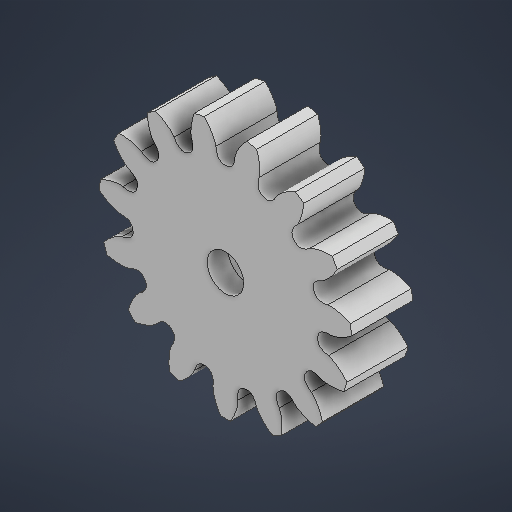
# Autodesk Inventor part: sg90 claw v2 gear m1
Saved by Autodesk Inventor 2026.1 (Build 301233020, 233B)
## iProperties
Created: 2025-05-11
Part Number: sg90 claw v2 gear m1
Material: Generic
Document SubType Name: Modeling
Designer: gavin
Density: 1 g/cm^3
Appearance: Default
Author: gavin
## iProperties of the stored document sg90 claw v2 gear m1_3D 列印.ipt
Created: 2025-05-11
Part Number: sg90 claw v2 gear m1_3D 列印
Material: 一般
Document SubType Name: Modeling
Designer: gavin
Density: 1 g/cm^3
Appearance: 預設
Author: gavin
Autodesk Inventor part; units mm, degrees
(part 1 of 2)
ref_plane "YZ Plane" through (0, 0, 0) normal (1, 0, 0) x (0, 1, 0)
ref_plane "XZ Plane" through (0, 0, 0) normal (0, 1, 0) x (-1, 0, 0)
ref_plane "XY Plane" through (0, 0, 0) normal (0, 0, 1) x (1, 0, 0)
sketch "Sketch1" plane through (0, 0, 0) normal (0, 0, 1) x (1, 0, 0)
  spline S0 degree 3 poles (-1.4265, 8.3497) (-1.3822, 8.3018) (-1.2937, 8.2061) (-1.1693, 8.0552) (-1.0517, 7.8988) (-0.9427, 7.7364) (-0.8433, 7.568) (-0.7701, 7.4222) (-0.7188, 7.3023) (-0.6849, 7.2106) (-0.6553, 7.1173) (-0.6433, 7.0532) (-0.6374, 7.0212) knots 0 0 0 0 0.125009 0.250019 0.375027 0.500033 0.625034 0.750026 0.812532 0.875035 0.937534 1 1 1 1
  spline S1 degree 3 poles (-0.6374, 7.0212) (-0.6343, 6.9735) (-0.6298, 6.9019) (-0.6162, 6.8071) (-0.6007, 6.7371) (-0.5816, 6.6679) (-0.5564, 6.6007) (-0.527, 6.5352) (-0.4905, 6.4733) (-0.4477, 6.4156) (-0.3983, 6.3633) (-0.3422, 6.3182) (-0.2804, 6.2814) (-0.2136, 6.2546) (-0.1435, 6.2382) (-0.0717, 6.2343) (0, 6.2359) (0.0717, 6.2343) (0.1435, 6.2382) (0.2136, 6.2546) (0.2804, 6.2814) (0.3422, 6.3182) (0.3983, 6.3633) (0.4477, 6.4156) (0.4905, 6.4733) (0.527, 6.5352) (0.5564, 6.6007) (0.5816, 6.6679) (0.6007, 6.7371) (0.6162, 6.8071) (0.6298, 6.9019) (0.6343, 6.9735) (0.6374, 7.0212) knots 0 0 0 0 0.062496 0.093751 0.125009 0.156269 0.187518 0.218773 0.250034 0.281288 0.312536 0.343783 0.375036 0.406281 0.437514 0.468742 0.5 0.531258 0.562486 0.593719 0.624964 0.656217 0.687464 0.718712 0.749966 0.781227 0.812482 0.843731 0.874991 0.906249 0.937504 1 1 1 1
  spline S2 degree 3 poles (0.6374, 7.0212) (0.6433, 7.0532) (0.6553, 7.1173) (0.6849, 7.2106) (0.7188, 7.3023) (0.7701, 7.4222) (0.8433, 7.568) (0.9427, 7.7364) (1.0517, 7.8988) (1.1693, 8.0552) (1.2937, 8.2061) (1.3822, 8.3018) (1.4265, 8.3497) knots 0 0 0 0 0.062466 0.124965 0.187468 0.249974 0.374966 0.499967 0.624973 0.749981 0.874991 1 1 1 1
  circle A0 centre (0, 0) radius 6.2354 construction
  circle A1 centre (0, 0) radius 7.0477 construction
  circle A2 centre (0, 0) radius 7.5 construction
  circle A3 centre (0, 0) radius 8.4706
  point P0 (-1.2951, 8.2049)
  point P1 (-1.1704, 8.0543)
  point P2 (-1.0532, 7.8978)
  point P3 (-0.9443, 7.7354)
  point P4 (-0.8452, 7.5669)
  point P5 (-0.7579, 7.392)
  point P6 (-0.7196, 7.302)
  point P7 (-0.6856, 7.2104)
  point P8 (-0.6572, 7.1168)
  point P9 (-0.6258, 6.8783)
  point P10 (-0.6153, 6.8073)
  point P11 (-0.6001, 6.7372)
  point P12 (-0.5806, 6.6682)
  point P13 (-0.5557, 6.6009)
  point P14 (-0.5258, 6.5358)
  point P15 (-0.4894, 6.4739)
  point P16 (-0.4466, 6.4165)
  point P17 (-0.3972, 6.3645)
  point P18 (-0.3413, 6.3196)
  point P19 (-0.2795, 6.2831)
  point P20 (-0.213, 6.2563)
  point P21 (-0.1432, 6.2403)
  point P22 (-0.0717, 6.2352)
  point P23 (0, 6.2354)
  point P24 (0.0717, 6.2352)
  point P25 (0.1432, 6.2403)
  point P26 (0.213, 6.2563)
  point P27 (0.2795, 6.2831)
  point P28 (0.3413, 6.3196)
  point P29 (0.3972, 6.3645)
  point P30 (0.4466, 6.4165)
  point P31 (0.4894, 6.4739)
  point P32 (0.5258, 6.5358)
  point P33 (0.5557, 6.6009)
  point P34 (0.5806, 6.6682)
  point P35 (0.6001, 6.7372)
  point P36 (0.6153, 6.8073)
  point P37 (0.6258, 6.8783)
  point P38 (0.6572, 7.1168)
  point P39 (0.6856, 7.2104)
  point P40 (0.7196, 7.302)
  point P41 (0.7579, 7.392)
  point P42 (0.8452, 7.5669)
  point P43 (0.9443, 7.7354)
  point P44 (1.0532, 7.8978)
  point P45 (1.1704, 8.0543)
  point P46 (1.2951, 8.2049)
  constraints: 4 centre point, 2 point on circle, 109 other
extrude "擠出1" add sketch "Sketch1" against normal blind 2.7
extrude "擠出2" cut sketch "Sketch1" against normal through all contours A3 S2 S1 S0 picked at (0.1465, 7.7452)
pattern_circular "環形陣列1" count 15 over 360 about axis through (0, 0, -10) along (0, 0, 1) of "擠出2"
sketch "草圖2" plane through (0, 0, 0) normal (0, 0, 1) x (1, 0, 0)
  circle A0 centre (0, 0) radius 2.2975
  dimension "d7" = 4.595
  constraints: 1 centre point, 1 coincident
  measures "d7" diameter of A0
extrude "擠出3" cut sketch "草圖2" against normal through all
sketch "草圖3" plane through (0, 0, 0) normal (0, 0, 1) x (1, 0, 0)
  circle A0 centre (0, 0) radius 2.2975 projected
  spline S0 degree 3 poles (4.6993, 7.0476) (4.6394, 7.0219) (4.5196, 6.9704) (4.3445, 6.8832) (4.1736, 6.7882) (4.0079, 6.6842) (3.8485, 6.5707) (3.7224, 6.4673) (3.6268, 6.3787) (3.5586, 6.3087) (3.4935, 6.2355) (3.4565, 6.1818) (3.438, 6.1549) knots 0 0 0 0 0.125009 0.250019 0.375027 0.500033 0.625034 0.750026 0.812532 0.875035 0.937534 1 1 1 1 projected
  spline S1 degree 3 poles (3.438, 6.1549) (3.4159, 6.1126) (3.3826, 6.049) (3.3316, 5.968) (3.289, 5.9103) (3.2434, 5.8548) (3.193, 5.8037) (3.1395, 5.7558) (3.081, 5.7141) (3.0184, 5.6788) (2.952, 5.6512) (2.8825, 5.6328) (2.811, 5.6244) (2.7391, 5.627) (2.6684, 5.6405) (2.6012, 5.6662) (2.5364, 5.6968) (2.4702, 5.7245) (2.4062, 5.7572) (2.3488, 5.8007) (2.2988, 5.8524) (2.2572, 5.9112) (2.2244, 5.9752) (2.2005, 6.043) (2.1848, 6.1131) (2.1766, 6.1845) (2.1764, 6.2563) (2.1807, 6.328) (2.1915, 6.3989) (2.2058, 6.4693) (2.2319, 6.5613) (2.2569, 6.6286) (2.2735, 6.6734) knots 0 0 0 0 0.062496 0.093751 0.125009 0.156269 0.187518 0.218773 0.250034 0.281288 0.312536 0.343783 0.375036 0.406281 0.437514 0.468742 0.5 0.531258 0.562486 0.593719 0.624964 0.656217 0.687464 0.718712 0.749966 0.781227 0.812482 0.843731 0.874991 0.906249 0.937504 1 1 1 1 projected
  spline S2 degree 3 poles (2.2735, 6.6734) (2.2811, 6.7051) (2.2963, 6.7685) (2.3071, 6.8658) (2.3135, 6.9634) (2.3154, 7.0938) (2.3078, 7.2567) (2.2855, 7.451) (2.2519, 7.6437) (2.2081, 7.8343) (2.1559, 8.0228) (2.1139, 8.1463) (2.093, 8.208) knots 0 0 0 0 0.062466 0.124965 0.187468 0.249974 0.374966 0.499967 0.624973 0.749981 0.874991 1 1 1 1 projected
  arc A1 (2.093, 8.208) -> (1.4265, 8.3497) centre (0, 0) ccw projected
  spline S3 degree 3 poles (1.4265, 8.3497) (1.3822, 8.3018) (1.2937, 8.2061) (1.1693, 8.0552) (1.0517, 7.8988) (0.9427, 7.7364) (0.8433, 7.568) (0.7701, 7.4222) (0.7188, 7.3023) (0.6849, 7.2106) (0.6553, 7.1173) (0.6433, 7.0532) (0.6374, 7.0212) knots 0 0 0 0 0.125009 0.250019 0.375027 0.500033 0.625034 0.750026 0.812532 0.875035 0.937534 1 1 1 1 projected
  spline S4 degree 3 poles (0.6374, 7.0212) (0.6343, 6.9735) (0.6298, 6.9019) (0.6162, 6.8071) (0.6007, 6.7371) (0.5816, 6.6679) (0.5564, 6.6007) (0.527, 6.5352) (0.4905, 6.4733) (0.4477, 6.4156) (0.3983, 6.3633) (0.3422, 6.3182) (0.2804, 6.2814) (0.2136, 6.2546) (0.1435, 6.2382) (0.0717, 6.2343) (0, 6.2359) (-0.0717, 6.2343) (-0.1435, 6.2382) (-0.2136, 6.2546) (-0.2804, 6.2814) (-0.3422, 6.3182) (-0.3983, 6.3633) (-0.4477, 6.4156) (-0.4905, 6.4733) (-0.527, 6.5352) (-0.5564, 6.6007) (-0.5816, 6.6679) (-0.6007, 6.7371) (-0.6162, 6.8071) (-0.6298, 6.9019) (-0.6343, 6.9735) (-0.6374, 7.0212) knots 0 0 0 0 0.062496 0.093751 0.125009 0.156269 0.187518 0.218773 0.250034 0.281288 0.312536 0.343783 0.375036 0.406281 0.437514 0.468742 0.5 0.531258 0.562486 0.593719 0.624964 0.656217 0.687464 0.718712 0.749966 0.781227 0.812482 0.843731 0.874991 0.906249 0.937504 1 1 1 1 projected
  spline S5 degree 3 poles (-0.6374, 7.0212) (-0.6433, 7.0532) (-0.6553, 7.1173) (-0.6849, 7.2106) (-0.7188, 7.3023) (-0.7701, 7.4222) (-0.8433, 7.568) (-0.9427, 7.7364) (-1.0517, 7.8988) (-1.1693, 8.0552) (-1.2937, 8.2061) (-1.3822, 8.3018) (-1.4265, 8.3497) knots 0 0 0 0 0.062466 0.124965 0.187468 0.249974 0.374966 0.499967 0.624973 0.749981 0.874991 1 1 1 1 projected
  arc A2 (-1.4265, 8.3497) -> (-2.093, 8.208) centre (0, 0) ccw projected
  spline S6 degree 3 poles (-2.093, 8.208) (-2.1139, 8.1463) (-2.1559, 8.0228) (-2.2081, 7.8343) (-2.2519, 7.6437) (-2.2855, 7.451) (-2.3078, 7.2567) (-2.3154, 7.0938) (-2.3135, 6.9634) (-2.3071, 6.8658) (-2.2963, 6.7685) (-2.2811, 6.7051) (-2.2735, 6.6734) knots 0 0 0 0 0.125009 0.250019 0.375027 0.500033 0.625034 0.750026 0.812532 0.875035 0.937534 1 1 1 1 projected
  spline S7 degree 3 poles (-2.2735, 6.6734) (-2.2569, 6.6286) (-2.2319, 6.5613) (-2.2058, 6.4693) (-2.1915, 6.3989) (-2.1807, 6.328) (-2.1764, 6.2563) (-2.1766, 6.1845) (-2.1848, 6.1131) (-2.2005, 6.043) (-2.2244, 5.9752) (-2.2572, 5.9112) (-2.2988, 5.8524) (-2.3488, 5.8007) (-2.4062, 5.7572) (-2.4702, 5.7245) (-2.5364, 5.6968) (-2.6012, 5.6662) (-2.6684, 5.6405) (-2.7391, 5.627) (-2.811, 5.6244) (-2.8825, 5.6328) (-2.952, 5.6512) (-3.0184, 5.6788) (-3.081, 5.7141) (-3.1395, 5.7558) (-3.193, 5.8037) (-3.2434, 5.8548) (-3.289, 5.9103) (-3.3316, 5.968) (-3.3826, 6.049) (-3.4159, 6.1126) (-3.438, 6.1549) knots 0 0 0 0 0.062496 0.093751 0.125009 0.156269 0.187518 0.218773 0.250034 0.281288 0.312536 0.343783 0.375036 0.406281 0.437514 0.468742 0.5 0.531258 0.562486 0.593719 0.624964 0.656217 0.687464 0.718712 0.749966 0.781227 0.812482 0.843731 0.874991 0.906249 0.937504 1 1 1 1 projected
  spline S8 degree 3 poles (-3.438, 6.1549) (-3.4565, 6.1818) (-3.4935, 6.2355) (-3.5586, 6.3087) (-3.6268, 6.3787) (-3.7224, 6.4673) (-3.8485, 6.5707) (-4.0079, 6.6842) (-4.1736, 6.7882) (-4.3445, 6.8832) (-4.5196, 6.9704) (-4.6394, 7.0219) (-4.6993, 7.0476) knots 0 0 0 0 0.062466 0.124965 0.187468 0.249974 0.374966 0.499967 0.624973 0.749981 0.874991 1 1 1 1 projected
  arc A3 (-4.6993, 7.0476) -> (-5.2505, 6.6471) centre (0, 0) ccw projected
  spline S9 degree 3 poles (-5.2505, 6.6471) (-5.2446, 6.5822) (-5.2327, 6.4524) (-5.2037, 6.2589) (-5.1662, 6.0669) (-5.1185, 5.8772) (-5.0598, 5.6906) (-5.0005, 5.5387) (-4.9457, 5.4204) (-4.9002, 5.3339) (-4.8508, 5.2494) (-4.8111, 5.1976) (-4.7913, 5.1717) knots 0 0 0 0 0.125009 0.250019 0.375027 0.500033 0.625034 0.750026 0.812532 0.875035 0.937534 1 1 1 1 projected
  spline S10 degree 3 poles (-4.7913, 5.1717) (-4.7578, 5.1376) (-4.7077, 5.0863) (-4.6464, 5.0128) (-4.6047, 4.9544) (-4.566, 4.8939) (-4.5329, 4.8302) (-4.5039, 4.7645) (-4.4824, 4.696) (-4.4681, 4.6255) (-4.4624, 4.5539) (-4.4663, 4.482) (-4.4804, 4.4115) (-4.5051, 4.3439) (-4.5399, 4.2808) (-4.585, 4.2248) (-4.6342, 4.1726) (-4.6809, 4.1183) (-4.7319, 4.0675) (-4.791, 4.0264) (-4.8556, 3.9948) (-4.9243, 3.9734) (-4.9954, 3.9619) (-5.0672, 3.9602) (-5.1388, 3.9669) (-5.2092, 3.9812) (-5.2776, 4.0032) (-5.3444, 4.0294) (-5.4086, 4.0616) (-5.471, 4.0969) (-5.5505, 4.1502) (-5.6067, 4.1947) (-5.6442, 4.2244) knots 0 0 0 0 0.062496 0.093751 0.125009 0.156269 0.187518 0.218773 0.250034 0.281288 0.312536 0.343783 0.375036 0.406281 0.437514 0.468742 0.5 0.531258 0.562486 0.593719 0.624964 0.656217 0.687464 0.718712 0.749966 0.781227 0.812482 0.843731 0.874991 0.906249 0.937504 1 1 1 1 projected
  spline S11 degree 3 poles (-5.6442, 4.2244) (-5.672, 4.2414) (-5.7277, 4.2755) (-5.8169, 4.3159) (-5.9077, 4.3521) (-6.0311, 4.3941) (-6.1884, 4.4373) (-6.3801, 4.4761) (-6.5737, 4.5038) (-6.7685, 4.521) (-6.964, 4.5295) (-7.0943, 4.5278) (-7.1595, 4.5269) knots 0 0 0 0 0.062466 0.124965 0.187468 0.249974 0.374966 0.499967 0.624973 0.749981 0.874991 1 1 1 1 projected
  arc A4 (-7.1595, 4.5269) -> (-7.5002, 3.9369) centre (0, 0) ccw projected
  spline S12 degree 3 poles (-7.5002, 3.9369) (-7.4684, 3.88) (-7.4047, 3.7662) (-7.2996, 3.6012) (-7.1872, 3.4411) (-7.0665, 3.2872) (-6.937, 3.1406) (-6.821, 3.026) (-6.7228, 2.9402) (-6.6461, 2.8796) (-6.5665, 2.8226) (-6.5092, 2.7914) (-6.4806, 2.7758) knots 0 0 0 0 0.125009 0.250019 0.375027 0.500033 0.625034 0.750026 0.812532 0.875035 0.937534 1 1 1 1 projected
  spline S13 degree 3 poles (-6.4806, 2.7758) (-6.4361, 2.7582) (-6.3694, 2.7318) (-6.2836, 2.6896) (-6.2217, 2.6532) (-6.1618, 2.6137) (-6.1057, 2.5689) (-6.0524, 2.5207) (-6.0049, 2.4668) (-5.9632, 2.4083) (-5.9288, 2.3451) (-5.9032, 2.2779) (-5.8874, 2.2077) (-5.8825, 2.1359) (-5.8885, 2.0642) (-5.907, 1.9947) (-5.9307, 1.927) (-5.9513, 1.8583) (-5.9772, 1.7912) (-6.0145, 1.7296) (-6.0606, 1.6744) (-6.1147, 1.6269) (-6.1749, 1.5876) (-6.2399, 1.5568) (-6.308, 1.5339) (-6.3782, 1.5182) (-6.4495, 1.5105) (-6.5213, 1.5073) (-6.593, 1.5106) (-6.6644, 1.5175) (-6.7587, 1.5338) (-6.8282, 1.5516) (-6.8745, 1.5635) knots 0 0 0 0 0.062496 0.093751 0.125009 0.156269 0.187518 0.218773 0.250034 0.281288 0.312536 0.343783 0.375036 0.406281 0.437514 0.468742 0.5 0.531258 0.562486 0.593719 0.624964 0.656217 0.687464 0.718712 0.749966 0.781227 0.812482 0.843731 0.874991 0.906249 0.937504 1 1 1 1 projected
  spline S14 degree 3 poles (-6.8745, 1.5635) (-6.9068, 1.5677) (-6.9715, 1.5762) (-7.0694, 1.5768) (-7.1671, 1.5729) (-7.2969, 1.5612) (-7.4581, 1.5366) (-7.6491, 1.4941) (-7.8372, 1.4406) (-8.0222, 1.3771) (-8.2042, 1.3054) (-8.3226, 1.2508) (-8.3818, 1.2235) knots 0 0 0 0 0.062466 0.124965 0.187468 0.249974 0.374966 0.499967 0.624973 0.749981 0.874991 1 1 1 1 projected
  arc A5 (-8.3818, 1.2235) -> (-8.453, 0.5459) centre (0, 0) ccw projected
  spline S15 degree 3 poles (-8.453, 0.5459) (-8.4008, 0.5069) (-8.2964, 0.4288) (-8.1333, 0.3209) (-7.9655, 0.2203) (-7.7926, 0.1289) (-7.6146, 0.0476) (-7.4621, -0.0099) (-7.3375, -0.0484) (-7.2427, -0.0725) (-7.1468, -0.0923) (-7.0818, -0.0975) (-7.0493, -0.1) knots 0 0 0 0 0.125009 0.250019 0.375027 0.500033 0.625034 0.750026 0.812532 0.875035 0.937534 1 1 1 1 projected
  spline S16 degree 3 poles (-7.0493, -0.1) (-7.0016, -0.0981) (-6.9299, -0.0951) (-6.8343, -0.0987) (-6.763, -0.1068) (-6.6921, -0.1185) (-6.6227, -0.1366) (-6.5544, -0.159) (-6.4891, -0.1888) (-6.4272, -0.2254) (-6.3701, -0.2691) (-6.3194, -0.3201) (-6.2763, -0.3778) (-6.2427, -0.4413) (-6.219, -0.5094) (-6.2076, -0.5804) (-6.2018, -0.6518) (-6.1927, -0.7229) (-6.189, -0.7948) (-6.198, -0.8662) (-6.2177, -0.9354) (-6.2478, -1.0008) (-6.2868, -1.0612) (-6.3336, -1.1158) (-6.3865, -1.1644) (-6.4443, -1.2072) (-6.5063, -1.2433) (-6.5705, -1.2754) (-6.6374, -1.3016) (-6.7054, -1.3244) (-6.7982, -1.3478) (-6.8689, -1.3598) (-6.9161, -1.3678) knots 0 0 0 0 0.062496 0.093751 0.125009 0.156269 0.187518 0.218773 0.250034 0.281288 0.312536 0.343783 0.375036 0.406281 0.437514 0.468742 0.5 0.531258 0.562486 0.593719 0.624964 0.656217 0.687464 0.718712 0.749966 0.781227 0.812482 0.843731 0.874991 0.906249 0.937504 1 1 1 1 projected
  spline S17 degree 3 poles (-6.9161, -1.3678) (-6.9473, -1.3771) (-7.0099, -1.3956) (-7.0995, -1.4349) (-7.1872, -1.4782) (-7.3011, -1.5417) (-7.4383, -1.6297) (-7.5955, -1.7462) (-7.7456, -1.8716) (-7.8888, -2.0049) (-8.0259, -2.1444) (-8.1118, -2.2424) (-8.1548, -2.2914) knots 0 0 0 0 0.062466 0.124965 0.187468 0.249974 0.374966 0.499967 0.624973 0.749981 0.874991 1 1 1 1 projected
  arc A6 (-8.1548, -2.2914) -> (-7.9443, -2.9395) centre (0, 0) ccw projected
  spline S18 degree 3 poles (-7.9443, -2.9395) (-7.8807, -2.9539) (-7.7535, -2.9827) (-7.5606, -3.015) (-7.3665, -3.0386) (-7.1713, -3.0518) (-6.9757, -3.0537) (-6.8129, -3.0442) (-6.6834, -3.0287) (-6.5871, -3.0121) (-6.4914, -2.9912) (-6.4299, -2.9695) (-6.3992, -2.9586) knots 0 0 0 0 0.125009 0.250019 0.375027 0.500033 0.625034 0.750026 0.812532 0.875035 0.937534 1 1 1 1 projected
  spline S19 degree 3 poles (-6.3992, -2.9586) (-6.3564, -2.9374) (-6.2921, -2.9055) (-6.2033, -2.8699) (-6.1348, -2.8483) (-6.0654, -2.8302) (-5.9945, -2.8185) (-5.9231, -2.8112) (-5.8512, -2.8119) (-5.7799, -2.8201) (-5.7099, -2.8368) (-5.6428, -2.8627) (-5.5801, -2.8979) (-5.5234, -2.9423) (-5.4742, -2.9948) (-5.4349, -3.0551) (-5.4005, -3.118) (-5.3632, -3.1792) (-5.3307, -3.2433) (-5.3098, -3.3123) (-5.2997, -3.3835) (-5.3006, -3.4555) (-5.3117, -3.5266) (-5.3322, -3.5955) (-5.3608, -3.6614) (-5.3961, -3.724) (-5.4381, -3.7822) (-5.4837, -3.8376) (-5.5341, -3.8887) (-5.5871, -3.9372) (-5.6623, -3.9964) (-5.722, -4.0361) (-5.7618, -4.0626) knots 0 0 0 0 0.062496 0.093751 0.125009 0.156269 0.187518 0.218773 0.250034 0.281288 0.312536 0.343783 0.375036 0.406281 0.437514 0.468742 0.5 0.531258 0.562486 0.593719 0.624964 0.656217 0.687464 0.718712 0.749966 0.781227 0.812482 0.843731 0.874991 0.906249 0.937504 1 1 1 1 projected
  spline S20 degree 3 poles (-5.7618, -4.0626) (-5.7866, -4.0838) (-5.8362, -4.1261) (-5.9021, -4.1985) (-5.9646, -4.2737) (-6.0428, -4.378) (-6.1324, -4.5143) (-6.2286, -4.6846) (-6.3147, -4.8603) (-6.3913, -5.0402) (-6.4598, -5.2234) (-6.4985, -5.3479) (-6.5178, -5.4102) knots 0 0 0 0 0.062466 0.124965 0.187468 0.249974 0.374966 0.499967 0.624973 0.749981 0.874991 1 1 1 1 projected
  arc A7 (-6.5178, -5.4102) -> (-6.0619, -5.9166) centre (0, 0) ccw projected
  spline S21 degree 3 poles (-6.0619, -5.9166) (-5.9979, -5.9039) (-5.8701, -5.8785) (-5.6807, -5.8295) (-5.4937, -5.7721) (-5.31, -5.7048) (-5.1306, -5.6269) (-4.9857, -5.552) (-4.8737, -5.4852) (-4.7924, -5.4309) (-4.7136, -5.3729) (-4.6662, -5.328) (-4.6426, -5.3056) knots 0 0 0 0 0.125009 0.250019 0.375027 0.500033 0.625034 0.750026 0.812532 0.875035 0.937534 1 1 1 1 projected
  spline S22 degree 3 poles (-4.6426, -5.3056) (-4.6121, -5.2688) (-4.5663, -5.2135) (-4.4997, -5.1449) (-4.4459, -5.0973) (-4.3898, -5.0525) (-4.3299, -5.013) (-4.2676, -4.9773) (-4.2017, -4.9487) (-4.1331, -4.9272) (-4.0625, -4.9139) (-3.9906, -4.9104) (-3.919, -4.917) (-3.8492, -4.9345) (-3.7828, -4.9625) (-3.7224, -5.0015) (-3.6654, -5.045) (-3.6064, -5.0858) (-3.5506, -5.1311) (-3.5035, -5.1856) (-3.4653, -5.2466) (-3.4369, -5.3127) (-3.4181, -5.3821) (-3.4088, -5.4534) (-3.4081, -5.5253) (-3.4149, -5.5968) (-3.4296, -5.6671) (-3.4487, -5.7363) (-3.474, -5.8035) (-3.5026, -5.8693) (-3.5473, -5.9539) (-3.5857, -6.0145) (-3.6113, -6.0549) knots 0 0 0 0 0.062496 0.093751 0.125009 0.156269 0.187518 0.218773 0.250034 0.281288 0.312536 0.343783 0.375036 0.406281 0.437514 0.468742 0.5 0.531258 0.562486 0.593719 0.624964 0.656217 0.687464 0.718712 0.749966 0.781227 0.812482 0.843731 0.874991 0.906249 0.937504 1 1 1 1 projected
  spline S23 degree 3 poles (-3.6113, -6.0549) (-3.6253, -6.0843) (-3.6534, -6.1432) (-3.6842, -6.2361) (-3.7107, -6.3302) (-3.7396, -6.4574) (-3.7661, -6.6183) (-3.7847, -6.813) (-3.7919, -7.0085) (-3.7887, -7.204) (-3.7768, -7.3993) (-3.7614, -7.5288) (-3.7538, -7.5935) knots 0 0 0 0 0.062466 0.124965 0.187468 0.249974 0.374966 0.499967 0.624973 0.749981 0.874991 1 1 1 1 projected
  arc A8 (-3.7538, -7.5935) -> (-3.1313, -7.8706) centre (0, 0) ccw projected
  spline S24 degree 3 poles (-3.1313, -7.8706) (-3.0781, -7.833) (-2.9716, -7.7578) (-2.8185, -7.636) (-2.671, -7.5076) (-2.5306, -7.3714) (-2.3983, -7.2272) (-2.2964, -7.0999) (-2.2213, -6.9933) (-2.1691, -6.9107) (-2.1207, -6.8256) (-2.0957, -6.7653) (-2.0832, -6.7352) knots 0 0 0 0 0.125009 0.250019 0.375027 0.500033 0.625034 0.750026 0.812532 0.875035 0.937534 1 1 1 1 projected
  spline S25 degree 3 poles (-2.0832, -6.7352) (-2.0703, -6.6892) (-2.051, -6.6201) (-2.018, -6.5303) (-1.9883, -6.465) (-1.9553, -6.4012) (-1.9166, -6.3407) (-1.8742, -6.2828) (-1.8256, -6.2298) (-1.7718, -6.1823) (-1.7126, -6.1415) (-1.6484, -6.109) (-1.5802, -6.0859) (-1.5093, -6.0735) (-1.4373, -6.072) (-1.3663, -6.0832) (-1.2965, -6.0997) (-1.2261, -6.113) (-1.1566, -6.1317) (-1.0915, -6.1623) (-1.0317, -6.2025) (-0.9789, -6.2513) (-0.9334, -6.3071) (-0.896, -6.3684) (-0.8661, -6.4338) (-0.8432, -6.5019) (-0.8281, -6.5721) (-0.8174, -6.6431) (-0.8132, -6.7147) (-0.8125, -6.7865) (-0.8189, -6.882) (-0.8294, -6.953) (-0.8363, -7.0003) knots 0 0 0 0 0.062496 0.093751 0.125009 0.156269 0.187518 0.218773 0.250034 0.281288 0.312536 0.343783 0.375036 0.406281 0.437514 0.468742 0.5 0.531258 0.562486 0.593719 0.624964 0.656217 0.687464 0.718712 0.749966 0.781227 0.812482 0.843731 0.874991 0.906249 0.937504 1 1 1 1 projected
  spline S26 degree 3 poles (-0.8363, -7.0003) (-0.8372, -7.0329) (-0.8388, -7.098) (-0.8292, -7.1955) (-0.8152, -7.2922) (-0.7899, -7.4201) (-0.7486, -7.5779) (-0.6864, -7.7634) (-0.6135, -7.9449) (-0.531, -8.1222) (-0.4407, -8.2958) (-0.374, -8.4078) (-0.3407, -8.4638) knots 0 0 0 0 0.062466 0.124965 0.187468 0.249974 0.374966 0.499967 0.624973 0.749981 0.874991 1 1 1 1 projected
  arc A9 (-0.3407, -8.4638) -> (0.3407, -8.4638) centre (0, 0) ccw projected
  spline S27 degree 3 poles (0.3407, -8.4638) (0.374, -8.4078) (0.4407, -8.2958) (0.531, -8.1222) (0.6135, -7.9449) (0.6864, -7.7634) (0.7486, -7.5779) (0.7899, -7.4201) (0.8152, -7.2922) (0.8292, -7.1955) (0.8388, -7.098) (0.8372, -7.0329) (0.8363, -7.0003) knots 0 0 0 0 0.125009 0.250019 0.375027 0.500033 0.625034 0.750026 0.812532 0.875035 0.937534 1 1 1 1 projected
  spline S28 degree 3 poles (0.8363, -7.0003) (0.8294, -6.953) (0.8189, -6.882) (0.8125, -6.7865) (0.8132, -6.7147) (0.8174, -6.6431) (0.8281, -6.5721) (0.8432, -6.5019) (0.8661, -6.4338) (0.896, -6.3684) (0.9334, -6.3071) (0.9789, -6.2513) (1.0317, -6.2025) (1.0915, -6.1623) (1.1566, -6.1317) (1.2261, -6.113) (1.2965, -6.0997) (1.3663, -6.0832) (1.4373, -6.072) (1.5093, -6.0735) (1.5802, -6.0859) (1.6484, -6.109) (1.7126, -6.1415) (1.7718, -6.1823) (1.8256, -6.2298) (1.8742, -6.2828) (1.9166, -6.3407) (1.9553, -6.4012) (1.9883, -6.465) (2.018, -6.5303) (2.051, -6.6201) (2.0703, -6.6892) (2.0832, -6.7352) knots 0 0 0 0 0.062496 0.093751 0.125009 0.156269 0.187518 0.218773 0.250034 0.281288 0.312536 0.343783 0.375036 0.406281 0.437514 0.468742 0.5 0.531258 0.562486 0.593719 0.624964 0.656217 0.687464 0.718712 0.749966 0.781227 0.812482 0.843731 0.874991 0.906249 0.937504 1 1 1 1 projected
  spline S29 degree 3 poles (2.0832, -6.7352) (2.0957, -6.7653) (2.1207, -6.8256) (2.1691, -6.9107) (2.2213, -6.9933) (2.2964, -7.0999) (2.3983, -7.2272) (2.5306, -7.3714) (2.671, -7.5076) (2.8185, -7.636) (2.9716, -7.7578) (3.0781, -7.833) (3.1313, -7.8706) knots 0 0 0 0 0.062466 0.124965 0.187468 0.249974 0.374966 0.499967 0.624973 0.749981 0.874991 1 1 1 1 projected
  arc A10 (3.1313, -7.8706) -> (3.7538, -7.5935) centre (0, 0) ccw projected
  spline S30 degree 3 poles (3.7538, -7.5935) (3.7614, -7.5288) (3.7768, -7.3993) (3.7887, -7.204) (3.7919, -7.0085) (3.7847, -6.813) (3.7661, -6.6183) (3.7396, -6.4574) (3.7107, -6.3302) (3.6842, -6.2361) (3.6534, -6.1432) (3.6253, -6.0843) (3.6113, -6.0549) knots 0 0 0 0 0.125009 0.250019 0.375027 0.500033 0.625034 0.750026 0.812532 0.875035 0.937534 1 1 1 1 projected
  spline S31 degree 3 poles (3.6113, -6.0549) (3.5857, -6.0145) (3.5473, -5.9539) (3.5026, -5.8693) (3.474, -5.8035) (3.4487, -5.7363) (3.4296, -5.6671) (3.4149, -5.5968) (3.4081, -5.5253) (3.4088, -5.4534) (3.4181, -5.3821) (3.4369, -5.3127) (3.4653, -5.2466) (3.5035, -5.1856) (3.5506, -5.1311) (3.6064, -5.0858) (3.6654, -5.045) (3.7224, -5.0015) (3.7828, -4.9625) (3.8492, -4.9345) (3.919, -4.917) (3.9906, -4.9104) (4.0625, -4.9139) (4.1331, -4.9272) (4.2017, -4.9487) (4.2676, -4.9773) (4.3299, -5.013) (4.3898, -5.0525) (4.4459, -5.0973) (4.4997, -5.1449) (4.5663, -5.2135) (4.6121, -5.2688) (4.6426, -5.3056) knots 0 0 0 0 0.062496 0.093751 0.125009 0.156269 0.187518 0.218773 0.250034 0.281288 0.312536 0.343783 0.375036 0.406281 0.437514 0.468742 0.5 0.531258 0.562486 0.593719 0.624964 0.656217 0.687464 0.718712 0.749966 0.781227 0.812482 0.843731 0.874991 0.906249 0.937504 1 1 1 1 projected
  spline S32 degree 3 poles (4.6426, -5.3056) (4.6662, -5.328) (4.7136, -5.3729) (4.7924, -5.4309) (4.8737, -5.4852) (4.9857, -5.552) (5.1306, -5.6269) (5.31, -5.7048) (5.4937, -5.7721) (5.6807, -5.8295) (5.8701, -5.8785) (5.9979, -5.9039) (6.0619, -5.9166) knots 0 0 0 0 0.062466 0.124965 0.187468 0.249974 0.374966 0.499967 0.624973 0.749981 0.874991 1 1 1 1 projected
  arc A11 (6.0619, -5.9166) -> (6.5178, -5.4102) centre (0, 0) ccw projected
  spline S33 degree 3 poles (6.5178, -5.4102) (6.4985, -5.3479) (6.4598, -5.2234) (6.3913, -5.0402) (6.3147, -4.8603) (6.2286, -4.6846) (6.1324, -4.5143) (6.0428, -4.378) (5.9646, -4.2737) (5.9021, -4.1985) (5.8362, -4.1261) (5.7866, -4.0838) (5.7618, -4.0626) knots 0 0 0 0 0.125009 0.250019 0.375027 0.500033 0.625034 0.750026 0.812532 0.875035 0.937534 1 1 1 1 projected
  spline S34 degree 3 poles (5.7618, -4.0626) (5.722, -4.0361) (5.6623, -3.9964) (5.5871, -3.9372) (5.5341, -3.8887) (5.4837, -3.8376) (5.4381, -3.7822) (5.3961, -3.724) (5.3608, -3.6614) (5.3322, -3.5955) (5.3117, -3.5266) (5.3006, -3.4555) (5.2997, -3.3835) (5.3098, -3.3123) (5.3307, -3.2433) (5.3632, -3.1792) (5.4005, -3.118) (5.4349, -3.0551) (5.4742, -2.9948) (5.5234, -2.9423) (5.5801, -2.8979) (5.6428, -2.8627) (5.7099, -2.8368) (5.7799, -2.8201) (5.8512, -2.8119) (5.9231, -2.8112) (5.9945, -2.8185) (6.0654, -2.8302) (6.1348, -2.8483) (6.2033, -2.8699) (6.2921, -2.9055) (6.3564, -2.9374) (6.3992, -2.9586) knots 0 0 0 0 0.062496 0.093751 0.125009 0.156269 0.187518 0.218773 0.250034 0.281288 0.312536 0.343783 0.375036 0.406281 0.437514 0.468742 0.5 0.531258 0.562486 0.593719 0.624964 0.656217 0.687464 0.718712 0.749966 0.781227 0.812482 0.843731 0.874991 0.906249 0.937504 1 1 1 1 projected
  spline S35 degree 3 poles (6.3992, -2.9586) (6.4299, -2.9695) (6.4914, -2.9912) (6.5871, -3.0121) (6.6834, -3.0287) (6.8129, -3.0442) (6.9757, -3.0537) (7.1713, -3.0518) (7.3665, -3.0386) (7.5606, -3.015) (7.7535, -2.9827) (7.8807, -2.9539) (7.9443, -2.9395) knots 0 0 0 0 0.062466 0.124965 0.187468 0.249974 0.374966 0.499967 0.624973 0.749981 0.874991 1 1 1 1 projected
  arc A12 (7.9443, -2.9395) -> (8.1548, -2.2914) centre (0, 0) ccw projected
  spline S36 degree 3 poles (8.1548, -2.2914) (8.1118, -2.2424) (8.0259, -2.1444) (7.8888, -2.0049) (7.7456, -1.8716) (7.5955, -1.7462) (7.4383, -1.6297) (7.3011, -1.5417) (7.1872, -1.4782) (7.0995, -1.4349) (7.0099, -1.3956) (6.9473, -1.3771) (6.9161, -1.3678) knots 0 0 0 0 0.125009 0.250019 0.375027 0.500033 0.625034 0.750026 0.812532 0.875035 0.937534 1 1 1 1 projected
  spline S37 degree 3 poles (6.9161, -1.3678) (6.8689, -1.3598) (6.7982, -1.3478) (6.7054, -1.3244) (6.6374, -1.3016) (6.5705, -1.2754) (6.5063, -1.2433) (6.4443, -1.2072) (6.3865, -1.1644) (6.3336, -1.1158) (6.2868, -1.0612) (6.2478, -1.0008) (6.2177, -0.9354) (6.198, -0.8662) (6.189, -0.7948) (6.1927, -0.7229) (6.2018, -0.6518) (6.2076, -0.5804) (6.219, -0.5094) (6.2427, -0.4413) (6.2763, -0.3778) (6.3194, -0.3201) (6.3701, -0.2691) (6.4272, -0.2254) (6.4891, -0.1888) (6.5544, -0.159) (6.6227, -0.1366) (6.6921, -0.1185) (6.763, -0.1068) (6.8343, -0.0987) (6.9299, -0.0951) (7.0016, -0.0981) (7.0493, -0.1) knots 0 0 0 0 0.062496 0.093751 0.125009 0.156269 0.187518 0.218773 0.250034 0.281288 0.312536 0.343783 0.375036 0.406281 0.437514 0.468742 0.5 0.531258 0.562486 0.593719 0.624964 0.656217 0.687464 0.718712 0.749966 0.781227 0.812482 0.843731 0.874991 0.906249 0.937504 1 1 1 1 projected
  spline S38 degree 3 poles (7.0493, -0.1) (7.0818, -0.0975) (7.1468, -0.0923) (7.2427, -0.0725) (7.3375, -0.0484) (7.4621, -0.0099) (7.6146, 0.0476) (7.7926, 0.1289) (7.9655, 0.2203) (8.1333, 0.3209) (8.2964, 0.4288) (8.4008, 0.5069) (8.453, 0.5459) knots 0 0 0 0 0.062466 0.124965 0.187468 0.249974 0.374966 0.499967 0.624973 0.749981 0.874991 1 1 1 1 projected
  arc A13 (8.453, 0.5459) -> (8.3818, 1.2235) centre (0, 0) ccw projected
  spline S39 degree 3 poles (8.3818, 1.2235) (8.3226, 1.2508) (8.2042, 1.3054) (8.0222, 1.3771) (7.8372, 1.4406) (7.6491, 1.4941) (7.4581, 1.5366) (7.2969, 1.5612) (7.1671, 1.5729) (7.0694, 1.5768) (6.9715, 1.5762) (6.9068, 1.5677) (6.8745, 1.5635) knots 0 0 0 0 0.125009 0.250019 0.375027 0.500033 0.625034 0.750026 0.812532 0.875035 0.937534 1 1 1 1 projected
  spline S40 degree 3 poles (6.8745, 1.5635) (6.8282, 1.5516) (6.7587, 1.5338) (6.6644, 1.5175) (6.593, 1.5106) (6.5213, 1.5073) (6.4495, 1.5105) (6.3782, 1.5182) (6.308, 1.5339) (6.2399, 1.5568) (6.1749, 1.5876) (6.1147, 1.6269) (6.0606, 1.6744) (6.0145, 1.7296) (5.9772, 1.7912) (5.9513, 1.8583) (5.9307, 1.927) (5.907, 1.9947) (5.8885, 2.0642) (5.8825, 2.1359) (5.8874, 2.2077) (5.9032, 2.2779) (5.9288, 2.3451) (5.9632, 2.4083) (6.0049, 2.4668) (6.0524, 2.5207) (6.1057, 2.5689) (6.1618, 2.6137) (6.2217, 2.6532) (6.2836, 2.6896) (6.3694, 2.7318) (6.4361, 2.7582) (6.4806, 2.7758) knots 0 0 0 0 0.062496 0.093751 0.125009 0.156269 0.187518 0.218773 0.250034 0.281288 0.312536 0.343783 0.375036 0.406281 0.437514 0.468742 0.5 0.531258 0.562486 0.593719 0.624964 0.656217 0.687464 0.718712 0.749966 0.781227 0.812482 0.843731 0.874991 0.906249 0.937504 1 1 1 1 projected
  spline S41 degree 3 poles (6.4806, 2.7758) (6.5092, 2.7914) (6.5665, 2.8226) (6.6461, 2.8796) (6.7228, 2.9402) (6.821, 3.026) (6.937, 3.1406) (7.0665, 3.2872) (7.1872, 3.4411) (7.2996, 3.6012) (7.4047, 3.7662) (7.4684, 3.88) (7.5002, 3.9369) knots 0 0 0 0 0.062466 0.124965 0.187468 0.249974 0.374966 0.499967 0.624973 0.749981 0.874991 1 1 1 1 projected
  arc A14 (7.5002, 3.9369) -> (7.1595, 4.5269) centre (0, 0) ccw projected
  spline S42 degree 3 poles (7.1595, 4.5269) (7.0943, 4.5278) (6.964, 4.5295) (6.7685, 4.521) (6.5737, 4.5038) (6.3801, 4.4761) (6.1884, 4.4373) (6.0311, 4.3941) (5.9077, 4.3521) (5.8169, 4.3159) (5.7277, 4.2755) (5.672, 4.2414) (5.6442, 4.2244) knots 0 0 0 0 0.125009 0.250019 0.375027 0.500033 0.625034 0.750026 0.812532 0.875035 0.937534 1 1 1 1 projected
  spline S43 degree 3 poles (5.6442, 4.2244) (5.6067, 4.1947) (5.5505, 4.1502) (5.471, 4.0969) (5.4086, 4.0616) (5.3444, 4.0294) (5.2776, 4.0032) (5.2092, 3.9812) (5.1388, 3.9669) (5.0672, 3.9602) (4.9954, 3.9619) (4.9243, 3.9734) (4.8556, 3.9948) (4.791, 4.0264) (4.7319, 4.0675) (4.6809, 4.1183) (4.6342, 4.1726) (4.585, 4.2248) (4.5399, 4.2808) (4.5051, 4.3439) (4.4804, 4.4115) (4.4663, 4.482) (4.4624, 4.5539) (4.4681, 4.6255) (4.4824, 4.696) (4.5039, 4.7645) (4.5329, 4.8302) (4.566, 4.8939) (4.6047, 4.9544) (4.6464, 5.0128) (4.7077, 5.0863) (4.7578, 5.1376) (4.7913, 5.1717) knots 0 0 0 0 0.062496 0.093751 0.125009 0.156269 0.187518 0.218773 0.250034 0.281288 0.312536 0.343783 0.375036 0.406281 0.437514 0.468742 0.5 0.531258 0.562486 0.593719 0.624964 0.656217 0.687464 0.718712 0.749966 0.781227 0.812482 0.843731 0.874991 0.906249 0.937504 1 1 1 1 projected
  spline S44 degree 3 poles (4.7913, 5.1717) (4.8111, 5.1976) (4.8508, 5.2494) (4.9002, 5.3339) (4.9457, 5.4204) (5.0005, 5.5387) (5.0598, 5.6906) (5.1185, 5.8772) (5.1662, 6.0669) (5.2037, 6.2589) (5.2327, 6.4524) (5.2446, 6.5822) (5.2505, 6.6471) knots 0 0 0 0 0.062466 0.124965 0.187468 0.249974 0.374966 0.499967 0.624973 0.749981 0.874991 1 1 1 1 projected
  arc A15 (5.2505, 6.6471) -> (4.6993, 7.0476) centre (0, 0) ccw projected
  constraints: 1 horizontal alignment, 44 other
extrude "擠出4" add sketch "草圖3" along normal blind 0.4 contours A0 | A15 S44 S43 S42 A14 S41 S40 S39 A13 S38 S37 S36 A12 S35 S34 S33 A11 S32 S31 S30 A10 S29 S28 S27 A9 S26 S25 S24 A8 S23 S22 S21 A7 S20 S19 S18 A6 S17 S16 S15 A5 S14 S13 S12 A4 S11 S10 S9 A3 S8 S7 S6 A2 S5 S4 S3 A1 S2 S1 S0
sketch "草圖4" plane through (0, 0, 0.4) normal (0, 0, 1) x (1, 0, 0)
  circle A0 centre (0, 0) radius 1.225
  dimension "d12" = 2.45
  constraints: 1 centre point, 1 coincident
  measures "d12" diameter of A0
extrude "擠出5" cut sketch "草圖4" against normal blind 3.104